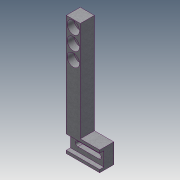
# Autodesk Inventor part: J005771
Saved by Autodesk Inventor 2015 SP1 (Build 190203100, 203)
## iProperties
Created: 2009-02-24
Part Number: J005771
Document SubType Name: Modeling
Designer: Ninglong Xu
Density: 7.8 g/cm^3
Material: STAINLESS STEEL, 17-4, H900
Mass: 11.8452 g
Surface Area: 64.0895 cm^2
Volume: 11.8452 cm^3
Description: MOUSE RIGHT HEADBAR BASE
Appearance: Metal-Steel (Stainless, Brushed)
Project: COMMON
Vendor: HHMI: JRC - ID&F
GlobalPropertyList: <PropertyList/>
ALTERED ITEM PART NUMBER: N/A
DESIGN DEPARTMENT: HHMI: JRC - ID&F
ALTERED ITEM DESCRIPTION: N/A
ALTERED ITEM VENDOR: N/A
SPECIAL FINISH: NONE
SURFACE ROUGHNESS: 63 Ra
LAB/DEPT: COMMON
REQUESTING SCIENTIST: COMMON
Revision Number: -
Autodesk Inventor part; units mm, degrees
note: some values were not read from the file. Chosen so that the rebuilt part matches the saved one: sketch regions of "Extrusion1".
ref_plane "YZ Plane" through (0, 0, 0) normal (1, 0, 0) x (0, 1, 0)
ref_plane "XZ Plane" through (0, 0, 0) normal (0, 1, 0) x (-1, 0, 0)
ref_plane "XY Plane" through (0, 0, 0) normal (0, 0, 1) x (1, 0, 0)
sketch "Sketch1" plane through (0, 0, 0) normal (0, 0, 1) x (1, 0, 0)
  line L0 (5.9388, 107.8209) -> (18.6388, 107.8209)
  line L1 (18.6388, 107.8209) -> (18.6388, -0.1291)
  line L2 (18.6388, -0.1291) -> (5.9388, -0.1291)
  line L3 (5.9388, -0.1291) -> (5.9388, 107.8209)
  line L4 (36.0759, 2.4109) -> (5.9388, 2.4109)
  line L5 (36.0759, 15.1363) -> (5.9388, 15.1363)
  line L6 (18.6388, -0.1291) -> (36.0759, -0.1291)
  line L7 (36.0759, -0.1291) -> (36.0759, 17.6763)
  line L8 (36.0759, 17.6763) -> (18.6388, 17.6763)
  circle A0 centre (31.6309, 8.7736) radius 2.159
  circle A1 centre (12.5809, 8.7736) radius 2.159
  line L9 (12.5809, 6.6146) -> (31.6309, 6.6146)
  line L10 (12.5809, 10.9326) -> (31.6309, 10.9326)
  point P0 (12.2762, 101.4709)
  point P1 (12.2762, 88.7709)
  point P2 (12.2762, 76.0709)
  point P3 (18.6388, 2.4109)
  point P4 (18.6388, 15.1363)
  dimension "d0" = 12.7
  dimension "d1" = 107.95
  dimension "d2" = 6.35
  dimension "d3" = 12.7
  dimension "d4" = 6.3626
  dimension "d5" = 6.3626
  dimension "d6" = 6.3626
  dimension "d7" = 12.7
  dimension "d8" = 2.54
  dimension "d9" = 12.7254
  dimension "d10" = 17.4371
  dimension "d11" = 2.54
  dimension "d12" = 4.318
  dimension "d13" = 6.3627
  dimension "d14" = 4.445
  dimension "d15" = 4.318
  dimension "d16" = 6.3627
  dimension "d17" = 19.05
  constraints: 22 end point, 9 point on line, 5 perpendicular, 4 parallel, 4 point on circle, 3 tangent, 2 centre point, 1 horizontal
  measures "d0" distance of L0.start L0.end
  measures "d1" distance of L0.end L1.end
  measures "d2" distance from line of L0 point (12.276, 101.471)
  measures "d3" distance of point (12.276, 88.771) point (12.276, 101.471)
  measures "d4" distance from line of L1 point (12.276, 101.471)
  measures "d5" distance from line of L1 point (12.276, 88.771)
  measures "d6" distance from line of L1 point (12.276, 76.071)
  measures "d7" distance of point (12.276, 76.071) point (12.276, 88.771)
  measures "d8" distance between parallel lines of L4 L2
  measures "d9" distance between parallel lines of L4 L5
  measures "d10" distance of L1.end L6.end
  measures "d11" distance between parallel lines of L5 L8
  measures "d12" diameter of A0
  measures "d13" distance from line of L4 A0.centre
  measures "d14" distance from line of L7 A0.centre
  measures "d15" diameter of A1
  measures "d16" distance from line of L4 A1.centre
  measures "d17" distance of A0.centre A1.centre
extrude "Extrusion1" add sketch "Sketch1" against normal blind 12.7 contours L0 L1 L5 L3 | L5 L1 L10 A1 L9 L4 L3 | L8 L7 L5 L1 | L4 L1 L2 L3 | L5 L7 L4 L1 L9 A0 L10 | L4 L7 L6 L1
extrude "Extrusion2" cut sketch "Sketch1" against normal blind 3.81 contours L5 L1 L10 A1 L9 L4 L3 | L5 L7 L4 L1 L9 A0 L10 | L1 L9 A1 L10
hole "Hole1" at (12.2762, 101.4709, 0) at (12.2762, 88.7709, 0) at (12.2762, 76.0709, 0) direction (0, 0, -1) diameter 6.5278 end through all counterbore diameter 11.1252 counterbore depth 6.35 clearance for "Socket Head Cap Screw" size "1/4" standard "Ansi Unified Screw Threads"
body "Solid1"
